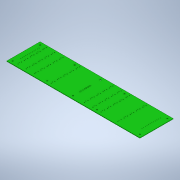
# Autodesk Inventor part: power_distro_pcb_RevC
Saved by Autodesk Inventor 2020.2 (Build 242310000, 310)
## iProperties
Created: 2019-11-25
Part Number: power_distro_pcb_RevC
Material: Nylon 6/6
Document SubType Name: Modeling
Designer: Rich
Density: 1.13 g/cm^3
Appearance: Dark Green
Author: Rich
Autodesk Inventor part; units mm, degrees
ref_plane "YZ Plane" through (0, 0, 0) normal (1, 0, 0) x (0, 1, 0)
ref_plane "XZ Plane" through (0, 0, 0) normal (0, 1, 0) x (-1, 0, 0)
ref_plane "XY Plane" through (0, 0, 0) normal (0, 0, 1) x (1, 0, 0)
sketch "Sketch2" plane through (0, 0, 0) normal (0, 1, 0) x (-1, 0, 0)
  circle A0 centre (127, 73.73) radius 1
  circle A1 centre (139.7, 8.89) radius 1.8986
  circle A2 centre (139.7, 92.71) radius 1.8986
  circle A3 centre (292.1, 8.89) radius 1.8986
  circle A4 centre (76.2, 82.48) radius 1
  circle A5 centre (76.2, 92.78) radius 1
  circle A6 centre (77.8, 87.63) radius 0.85
  circle A7 centre (76.2, 63.43) radius 1
  circle A8 centre (76.2, 73.73) radius 1
  circle A9 centre (77.8, 68.58) radius 0.85
  circle A10 centre (76.2, 44.38) radius 1
  circle A11 centre (76.2, 54.68) radius 1
  circle A12 centre (77.8, 49.53) radius 0.85
  circle A13 centre (76.2, 25.33) radius 1
  circle A14 centre (76.2, 35.63) radius 1
  circle A15 centre (77.8, 30.48) radius 0.85
  circle A16 centre (279.4, 6.28) radius 1
  circle A17 centre (279.4, 16.58) radius 1
  circle A18 centre (281, 11.43) radius 0.85
  circle A19 centre (127, 82.48) radius 1
  circle A20 centre (127, 92.78) radius 1
  circle A21 centre (128.6, 87.63) radius 0.85
  circle A22 centre (127, 63.43) radius 1
  circle A23 centre (355.6, 6.28) radius 1
  circle A24 centre (128.6, 68.58) radius 0.85
  circle A25 centre (127, 44.38) radius 1
  circle A26 centre (127, 54.68) radius 1
  circle A27 centre (128.6, 49.53) radius 0.85
  circle A28 centre (127, 25.33) radius 1
  circle A29 centre (127, 35.63) radius 1
  circle A30 centre (128.6, 30.48) radius 0.85
  circle A31 centre (330.2, 6.28) radius 1
  circle A32 centre (330.2, 16.58) radius 1
  circle A33 centre (331.8, 11.43) radius 0.85
  circle A34 centre (152.4, 82.48) radius 1
  circle A35 centre (152.4, 92.78) radius 1
  circle A36 centre (154, 87.63) radius 0.85
  circle A37 centre (152.4, 63.43) radius 1
  circle A38 centre (152.4, 73.73) radius 1
  circle A39 centre (154, 68.58) radius 0.85
  circle A40 centre (152.4, 44.38) radius 1
  circle A41 centre (152.4, 54.68) radius 1
  circle A42 centre (154, 49.53) radius 0.85
  circle A43 centre (152.4, 25.33) radius 1
  circle A44 centre (152.4, 35.63) radius 1
  circle A45 centre (154, 30.48) radius 0.85
  circle A46 centre (292.1, 92.71) radius 1.8986
  circle A47 centre (355.6, 16.58) radius 1
  circle A48 centre (357.2, 11.43) radius 0.85
  circle A49 centre (177.8, 82.48) radius 1
  circle A50 centre (177.8, 92.78) radius 1
  circle A51 centre (179.4, 87.63) radius 0.85
  circle A52 centre (177.8, 63.43) radius 1
  circle A53 centre (177.8, 73.73) radius 1
  circle A54 centre (179.4, 68.58) radius 0.85
  circle A55 centre (177.8, 44.38) radius 1
  circle A56 centre (177.8, 54.68) radius 1
  circle A57 centre (179.4, 49.53) radius 0.85
  circle A58 centre (177.8, 25.33) radius 1
  circle A59 centre (177.8, 35.63) radius 1
  circle A60 centre (179.4, 30.48) radius 0.85
  circle A61 centre (381, 6.28) radius 1
  circle A62 centre (381, 16.58) radius 1
  circle A63 centre (382.6, 11.43) radius 0.85
  circle A64 centre (76.2, 6.28) radius 1
  circle A65 centre (76.2, 16.58) radius 1
  circle A66 centre (77.8, 11.43) radius 0.85
  circle A67 centre (127, 6.28) radius 1
  circle A68 centre (127, 16.58) radius 1
  circle A69 centre (128.6, 11.43) radius 0.85
  circle A70 centre (152.4, 6.28) radius 1
  circle A71 centre (152.4, 16.58) radius 1
  circle A72 centre (154, 11.43) radius 0.85
  circle A73 centre (177.8, 6.28) radius 1
  circle A74 centre (177.8, 16.58) radius 1
  circle A75 centre (179.4, 11.43) radius 0.85
  circle A76 centre (279.4, 25.33) radius 1
  circle A77 centre (279.4, 35.63) radius 1
  circle A78 centre (281, 30.48) radius 0.85
  circle A79 centre (330.2, 25.33) radius 1
  circle A80 centre (330.2, 35.63) radius 1
  circle A81 centre (331.8, 30.48) radius 0.85
  circle A82 centre (355.6, 25.33) radius 1
  circle A83 centre (355.6, 35.63) radius 1
  circle A84 centre (357.2, 30.48) radius 0.85
  circle A85 centre (381, 25.33) radius 1
  circle A86 centre (381, 35.63) radius 1
  circle A87 centre (382.6, 30.48) radius 0.85
  circle A88 centre (279.4, 44.38) radius 1
  circle A89 centre (279.4, 54.68) radius 1
  circle A90 centre (281, 49.53) radius 0.85
  circle A91 centre (330.2, 44.38) radius 1
  circle A92 centre (330.2, 54.68) radius 1
  circle A93 centre (331.8, 49.53) radius 0.85
  circle A94 centre (355.6, 44.38) radius 1
  circle A95 centre (355.6, 54.68) radius 1
  circle A96 centre (357.2, 49.53) radius 0.85
  circle A97 centre (381, 44.38) radius 1
  circle A98 centre (381, 54.68) radius 1
  circle A99 centre (382.6, 49.53) radius 0.85
  circle A100 centre (279.4, 82.48) radius 1
  circle A101 centre (279.4, 92.78) radius 1
  circle A102 centre (281, 87.63) radius 0.85
  circle A103 centre (330.2, 82.48) radius 1
  circle A104 centre (330.2, 92.78) radius 1
  circle A105 centre (331.8, 87.63) radius 0.85
  circle A106 centre (355.6, 82.48) radius 1
  circle A107 centre (355.6, 92.78) radius 1
  circle A108 centre (357.2, 87.63) radius 0.85
  circle A109 centre (381, 82.48) radius 1
  circle A110 centre (381, 92.78) radius 1
  circle A111 centre (382.6, 87.63) radius 0.85
  circle A112 centre (279.4, 63.43) radius 1
  circle A113 centre (279.4, 73.73) radius 1
  circle A114 centre (281, 68.58) radius 0.85
  circle A115 centre (330.2, 63.43) radius 1
  circle A116 centre (330.2, 73.73) radius 1
  circle A117 centre (331.8, 68.58) radius 0.85
  circle A118 centre (355.6, 63.43) radius 1
  circle A119 centre (355.6, 73.73) radius 1
  circle A120 centre (357.2, 68.58) radius 0.85
  circle A121 centre (381, 63.43) radius 1
  circle A122 centre (381, 73.73) radius 1
  circle A123 centre (382.6, 68.58) radius 0.85
  circle A124 centre (212.09, 72.39) radius 0.4953
  circle A125 centre (214.63, 72.39) radius 0.4953
  circle A126 centre (212.09, 69.85) radius 0.4953
  circle A127 centre (214.63, 69.85) radius 0.4953
  circle A128 centre (212.09, 67.31) radius 0.4953
  circle A129 centre (214.63, 67.31) radius 0.4953
  circle A130 centre (212.09, 64.77) radius 0.4953
  circle A131 centre (214.63, 64.77) radius 0.4953
  circle A132 centre (212.09, 62.23) radius 0.4953
  circle A133 centre (214.63, 62.23) radius 0.4953
  circle A134 centre (212.09, 59.69) radius 0.4953
  circle A135 centre (214.63, 59.69) radius 0.4953
  circle A136 centre (212.09, 57.15) radius 0.4953
  circle A137 centre (214.63, 57.15) radius 0.4953
  circle A138 centre (212.09, 54.61) radius 0.4953
  circle A139 centre (214.63, 54.61) radius 0.4953
  circle A140 centre (212.09, 52.07) radius 0.4953
  circle A141 centre (214.63, 52.07) radius 0.4953
  circle A142 centre (212.09, 49.53) radius 0.4953
  circle A143 centre (214.63, 49.53) radius 0.4953
  circle A144 centre (212.09, 46.99) radius 0.4953
  circle A145 centre (214.63, 46.99) radius 0.4953
  circle A146 centre (212.09, 44.45) radius 0.4953
  circle A147 centre (214.63, 44.45) radius 0.4953
  circle A148 centre (212.09, 41.91) radius 0.4953
  circle A149 centre (214.63, 41.91) radius 0.4953
  circle A150 centre (212.09, 39.37) radius 0.4953
  circle A151 centre (214.63, 39.37) radius 0.4953
  circle A152 centre (21, 74.315) radius 0.7
  circle A153 centre (21, 69.235) radius 0.7
  circle A154 centre (21, 64.155) radius 0.7
  circle A155 centre (21, 59.075) radius 0.7
  circle A156 centre (21, 53.995) radius 0.7
  circle A157 centre (21, 48.915) radius 0.7
  circle A158 centre (21, 43.835) radius 0.7
  circle A159 centre (21, 38.755) radius 0.7
  circle A160 centre (21, 33.675) radius 0.7
  circle A161 centre (21, 28.595) radius 0.7
  circle A162 centre (21, 23.515) radius 0.7
  circle A163 centre (21, 18.435) radius 0.7
  circle A164 centre (391.125, 18.435) radius 0.7
  circle A165 centre (391.125, 23.515) radius 0.7
  circle A166 centre (391.125, 28.595) radius 0.7
  circle A167 centre (391.125, 33.675) radius 0.7
  circle A168 centre (391.125, 38.755) radius 0.7
  circle A169 centre (391.125, 43.835) radius 0.7
  circle A170 centre (391.125, 48.915) radius 0.7
  circle A171 centre (391.125, 53.995) radius 0.7
  circle A172 centre (391.125, 59.075) radius 0.7
  circle A173 centre (391.125, 64.155) radius 0.7
  circle A174 centre (391.125, 69.235) radius 0.7
  circle A175 centre (391.125, 74.315) radius 0.7
  circle A176 centre (8.89, 8.89) radius 1.8986
  circle A177 centre (397.51, 92.71) radius 1.8986
  circle A178 centre (397.51, 8.89) radius 1.8986
  circle A179 centre (8.89, 92.71) radius 1.8986
  circle A180 centre (213.36, 92.71) radius 1.8986
  circle A181 centre (213.36, 8.89) radius 1.8986
  line L0 (406.4, 0) -> (406.4, 101.6)
  line L1 (406.4, 101.6) -> (0, 101.6)
  line L2 (0, 101.6) -> (0, 0)
  line L3 (0, 0) -> (406.4, 0)
  constraints: 182 centre point, 8 end point
extrude "Extrusion2" add sketch "Sketch2" against normal blind 1.5748
body "Solid2"
